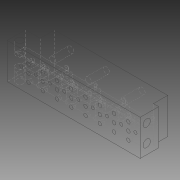
# Autodesk Inventor part: ValveManifold shared no and nc individual common
Saved by Autodesk Inventor 2011 (Build 150239000, 239)
## iProperties
Created: 2012-03-09
Part Number: ValveManifold shared no and nc individual common
Document SubType Name: Modeling
Designer: Marc
Density: 1 g/cm^3
Author: Marc
Autodesk Inventor part; units mm, degrees
ref_plane "YZ Plane" through (0, 0, 0) normal (1, 0, 0) x (0, 1, 0)
ref_plane "XZ Plane" through (0, 0, 0) normal (0, 1, 0) x (-1, 0, 0)
sketch "Sketch1" plane through (0, 0, 0) normal (0, 0, 1) x (1, 0, 0)
  line L0 (0, 0) -> (71.12, 0)
  line L1 (71.12, 0) -> (71.12, 19.05)
  line L2 (71.12, 19.05) -> (0, 19.05)
  line L3 (0, 19.05) -> (0, 0)
  dimension "ManifoldWidth" = 71.12
  dimension "ManifoldDepth" = 19.05
  constraints: 8 end point, 2 parallel, 1 horizontal, 1 perpendicular
  measures "ManifoldWidth" distance of L0.start L0.end
  measures "ManifoldDepth" distance of L0.end L1.end
extrude "Extrusion1" add sketch "Sketch1" along normal blind 17.4625
sketch "hdi facemount placement" plane through (0, 0, 17.4625) normal (0, 0, 1) x (1, 0, 0)
  line L0 (0, 0) -> (0, 19.05) projected
  line L1 (71.12, 0) -> (0, 0) projected
  line L2 (71.12, 19.05) -> (71.12, 0) projected
  line L3 (0, 19.05) -> (71.12, 19.05) projected
  line L4 (11.43, 13.7668) -> (11.43, 5.2832)
  line L5 (7.62, 10.7442) -> (15.24, 10.7442)
  line L6 (35.56, 19.05) -> (35.56, 0)
  line L7 (0, 9.525) -> (71.12, 9.525)
  point P0 (11.43, 9.525)
  point P1 (19.05, 5.2832)
  point P2 (22.86, 10.7442)
  point P3 (19.05, 13.7668)
  point P4 (19.05, 9.525)
  point P5 (26.67, 5.2832)
  point P6 (30.48, 10.7442)
  point P7 (26.67, 13.7668)
  point P8 (26.67, 9.525)
  point P9 (34.29, 5.2832)
  point P10 (38.1, 10.7442)
  point P11 (34.29, 13.7668)
  point P12 (34.29, 9.525)
  point P13 (41.91, 5.2832)
  point P14 (45.72, 10.7442)
  point P15 (41.91, 13.7668)
  point P16 (41.91, 9.525)
  point P17 (49.53, 5.2832)
  point P18 (53.34, 10.7442)
  point P19 (49.53, 13.7668)
  point P20 (49.53, 9.525)
  point P21 (57.15, 5.2832)
  point P22 (60.96, 10.7442)
  point P23 (57.15, 13.7668)
  point P24 (57.15, 9.525)
  point P25 (64.77, 5.2832)
  point P26 (68.58, 10.7442)
  point P27 (64.77, 13.7668)
  point P28 (64.77, 9.525)
  dimension "d4" = 8.4836
  dimension "d5" = 7.62
  dimension "d6" = 3.0226
  dimension "d7" = 1.2192
  dimension "d10" = 7.62
  dimension "d106" = 5.2832
  dimension "d160" = 7.62
  constraints: 8 end point, 5 midpoint, 4 coincident, 2 perpendicular, 1 horizontal, 1 point on line, 1 symmetric about line, 28 other
  measures "d4" distance of L4.start L4.end
  measures "d5" distance of L5.start L5.end
  measures "d6" vertical distance of L4.start L5.end
  measures "d7" distance from line of L5 point (11.43, 9.525)
  measures "d10" distance of point (11.43, 13.767) point (19.05, 13.767)
  measures "d106" distance from line of L3 L4.start
  measures "d160" distance from line of L0 L5.start
hole "facemount tapped holes" at (7.62, 10.7442, 17.4625) at (15.24, 10.7442, 17.4625) at (22.86, 10.7442, 17.4625) at (30.48, 10.7442, 17.4625) at (38.1, 10.7442, 17.4625) at (45.72, 10.7442, 17.4625) at (53.34, 10.7442, 17.4625) at (60.96, 10.7442, 17.4625) at (68.58, 10.7442, 17.4625) direction (0, 0, -1) diameter 1.7018 depth 6.35 tip angle 118
hole "normally open holes" at (11.43, 13.7668, 17.4625) at (19.05, 13.7668, 17.4625) at (26.67, 13.7668, 17.4625) at (34.29, 13.7668, 17.4625) at (41.91, 13.7668, 17.4625) at (49.53, 13.7668, 17.4625) at (57.15, 13.7668, 17.4625) at (64.77, 13.7668, 17.4625) direction (0, 0, -1) diameter 1.9304 depth 3.4417 tip angle 118
hole "normally closed holes" at (11.43, 5.2832, 17.4625) at (19.05, 5.2832, 17.4625) at (26.67, 5.2832, 17.4625) at (34.29, 5.2832, 17.4625) at (41.91, 5.2832, 17.4625) at (49.53, 5.2832, 17.4625) at (57.15, 5.2832, 17.4625) at (64.77, 5.2832, 17.4625) direction (0, 0, -1) diameter 1.9304 depth 3.4417 tip angle 118
hole "shallow common holes" at (11.43, 9.525, 17.4625) at (26.67, 9.525, 17.4625) at (41.91, 9.525, 17.4625) at (57.15, 9.525, 17.4625) direction (0, 0, -1) diameter 1.9304 depth 7.9375 tip angle 118
hole "deep common holes" at (19.05, 9.525, 17.4625) at (34.29, 9.525, 17.4625) at (49.53, 9.525, 17.4625) at (64.77, 9.525, 17.4625) direction (0, 0, -1) diameter 1.9304 depth 13.0175 tip angle 118
sketch "Sketch3" plane through (71.12, 0, 0) normal (1, 0, 0) x (0, 0, -1)
  line L0 (-17.4625, 12.8016) -> (-17.4625, 14.732) projected
  line L1 (0, 0) -> (-17.4625, 0) projected
  line L2 (-17.4625, 0) -> (-17.4625, 19.05) projected
  line L3 (-17.4625, 19.05) -> (0, 19.05) projected
  line L4 (0, 19.05) -> (0, 0) projected
  line L5 (0, 0) -> (-17.4625, 0) projected
  line L6 (-17.4625, 0) -> (-17.4625, 19.05) projected
  line L7 (-17.4625, 19.05) -> (0, 19.05) projected
  line L8 (0, 19.05) -> (0, 0) projected
  line L9 (-14.0208, 14.732) -> (-14.0208, 12.8016) projected
  line L10 (-14.0208, 12.8016) -> (-17.4625, 12.8016) projected
  line L11 (-14.0208, 14.732) -> (-17.4625, 14.732) projected
  line L12 (-14.0208, 6.2484) -> (-17.4625, 6.2484) projected
  line L13 (-14.0208, 4.318) -> (-17.4625, 4.318) projected
  line L14 (-14.0208, 6.2484) -> (-14.0208, 4.318) projected
  line L15 (-11.1125, 11.5951) -> (-17.4625, 11.5951) projected
  line L16 (-10.8458, 7.1163) -> (-10.8458, 3.4501)
  line L17 (-10.8458, 3.4501) -> (-14.0208, 1.617)
  line L18 (-14.0208, 1.617) -> (-17.1958, 3.4501)
  line L19 (-17.1958, 3.4501) -> (-17.1958, 7.1163)
  line L20 (-17.1958, 7.1163) -> (-14.0208, 8.9494)
  line L21 (-14.0208, 8.9494) -> (-10.8458, 7.1163)
  circle A0 centre (-14.0208, 5.2832) radius 3.6662
  line L22 (-10.8458, 16.5651) -> (-10.8458, 12.8989)
  line L23 (-10.8458, 12.8989) -> (-14.0208, 11.0658)
  line L24 (-14.0208, 11.0658) -> (-17.1958, 12.8989)
  line L25 (-17.1958, 12.8989) -> (-17.1958, 16.5651)
  line L26 (-17.1958, 16.5651) -> (-14.0208, 18.3982)
  line L27 (-14.0208, 18.3982) -> (-10.8458, 16.5651)
  circle A1 centre (-14.0208, 14.732) radius 3.6662
  point P0 (-17.4625, 13.7668)
  dimension "d44" = 3.1369
  dimension "d121" = 5.2832
  dimension "d122" = 4.318
  dimension "d161" = 6.35
  dimension "d162" = 9.4488
  constraints: 24 end point, 6 coincident, 2 collinear, 2 vertical alignment, 1 midpoint, 1 parallel, 30 other
  measures "d44" distance from line of L15 L9.start
  measures "d121" distance from line of L1 point (-14.021, 5.283)
  measures "d122" distance from line of L3 L9.start
  measures "d161" distance between parallel lines of L17 L20
  measures "d162" distance of point (-14.021, 14.732) point (-14.021, 5.283)
hole "shared reservoirs" at (71.12, 5.2832, 14.0208) at (71.12, 14.732, 14.0208) direction (-1, 0, 0) diameter 3.9624 depth 67.945 tip angle 118 thread size "10-32 UNF" class "2B" standard "ANSI Unified Screw Threads"
sketch "Sketch6" plane through (0, 0, 0) normal (0, 0, -1) x (-1, 0, 0)
  line L0 (-71.12, 19.05) -> (0, 19.05) projected
  arc A0 (-26.67, 12.8016) -> (-26.67, 12.8016) centre (-26.67, 12.8016) ccw projected
  line L1 (-3.175, 16.7132) -> (-71.12, 16.7132) projected
  arc A1 (-26.67, 4.318) -> (-26.67, 4.318) centre (-26.67, 4.318) ccw projected
  line L2 (-3.175, 3.302) -> (-71.12, 3.302) projected
  line L3 (-3.175, 12.7508) -> (-71.12, 12.7508) projected
  circle A2 centre (-30.48, 10.7442) radius 0.8509 projected
  circle A3 centre (-22.86, 10.7442) radius 0.8509 projected
  line L4 (-35.56, 19.05) -> (-35.56, 0) projected
  point P0 (-16.51, 14.2875)
  point P1 (-35.56, 14.2875)
  point P2 (-54.61, 14.2875)
  dimension "d82" = 19.05
  dimension "d87" = 4.7625
  constraints: 1 horizontal, 1 symmetric about line, 4 other
  measures "d82" distance of point (-16.51, 14.287) point (-35.56, 14.287)
  measures "d87" distance from line of L0 point (-16.51, 14.287)
hole "8-32 mounting holes" at (16.51, 14.2875, 0) at (35.56, 14.2875, 0) at (54.61, 14.2875, 0) direction (0, 0, 1) diameter 3.302 depth 9.525 tip angle 118 thread size "8-32 UNC" class "2B" standard "ANSI Unified Screw Threads"
sketch "Sketch9" plane through (0, 19.05, 0) normal (0, 1, 0) x (1, 0, 0)
  line L0 (71.12, 0) -> (71.12, -17.4625) projected
  line L1 (0, 0) -> (0, -17.4625) projected
  line L2 (6.7691, -11.1125) -> (6.7691, -17.4625) projected
  line L3 (3.175, -12.0396) -> (71.12, -12.0396) projected
  line L4 (3.175, -16.002) -> (71.12, -16.002) projected
  line L5 (3.175, -16.002) -> (3.175, -12.0396)
  line L6 (71.12, -16.002) -> (71.12, -12.0396)
  line L7 (71.12, -14.0208) -> (3.175, -14.0208) construction
  circle A0 centre (3.3846, -14.0208) radius 3.3846
  point P0 (0, -17.4625)
  constraints: 6 end point, 2 midpoint, 1 centre point, 1 coincident, 1 collinear, 1 perpendicular, 1 point on line, 1 tangent, 2 other
hole "normally open connection 2" at (3.3845, 19.05, 14.0208) direction (0, -1, 0) diameter 3.9624 depth 6.35 tip angle 118 thread size "10-32 UNF" class "2B" standard "ANSI Unified Screw Threads"
sketch "Sketch10" plane through (0, 0, 0) normal (0, -1, 0) x (1, 0, 0)
  circle A0 centre (3.3845, 14.0208) radius 1.9812 projected
  line L0 (8.9408, 10.8129) -> (3.3845, 7.605)
  line L1 (3.3845, 7.605) -> (-2.1717, 10.8129)
  line L2 (-2.1717, 10.8129) -> (-2.1717, 17.2287)
  line L3 (-2.1717, 17.2287) -> (3.3845, 20.4366)
  line L4 (3.3845, 20.4366) -> (8.9408, 17.2287)
  line L5 (8.9408, 17.2287) -> (8.9408, 10.8129)
  circle A1 centre (3.3845, 14.0208) radius 6.4158
  dimension "d158" = 11.1125
  constraints: 12 end point, 3 coincident, 1 vertical, 16 other
  measures "d158" distance between parallel lines of L5 L2
hole "normally closed connection 2" at (3.3845, 0, 14.0208) direction (0, 1, 0) diameter 3.9624 depth 7.112 tip angle 118 thread size "10-32 UNF" class "2B" standard "ANSI Unified Screw Threads"
sketch "Sketch11" plane through (0, 0, 0) normal (0, -1, 0) x (1, 0, 0)
  line L0 (71.12, 17.4625) -> (0, 17.4625) projected
  line L1 (12.3952, 9.525) -> (12.3952, 17.4625) projected
  line L2 (10.4648, 9.525) -> (10.4648, 17.4625) projected
  line L3 (18.0848, 4.445) -> (18.0848, 17.4625) projected
  line L4 (20.0152, 4.445) -> (20.0152, 17.4625) projected
  line L5 (12.3952, 9.525) -> (10.4648, 9.525) projected
  line L6 (20.0152, 4.445) -> (18.0848, 4.445) projected
  circle A0 centre (11.43, 9.525) radius 3.175
  point P0 (19.05, 4.445)
  point P1 (26.67, 9.525)
  point P2 (34.29, 4.445)
  point P3 (41.91, 9.525)
  point P4 (49.53, 4.445)
  point P5 (57.15, 9.525)
  point P6 (64.77, 4.445)
  dimension "d139" = 15.24
  dimension "d159" = 6.35
  constraints: 2 midpoint, 1 centre point, 1 coincident, 1 horizontal, 6 other
  measures "d139" distance of point (11.43, 9.525) point (26.67, 9.525)
  measures "d159" diameter of A0
ref_plane "Work Plane1" through (11.43, 9.525, 17.4625) normal (0, -1, 0) x (1, 0, 0)
hole "Hole15" at (11.43, 0, 9.525) at (19.05, 0, 4.445) at (26.67, 0, 9.525) at (34.29, 0, 4.445) at (41.91, 0, 9.525) at (49.53, 0, 4.445) at (57.15, 0, 9.525) at (64.77, 0, 4.445) direction (0, 1, 0) diameter 1.016 depth 9.525
hole "Hole16" at (11.43, 0, 9.525) at (19.05, 0, 4.445) at (26.67, 0, 9.525) at (34.29, 0, 4.445) at (41.91, 0, 9.525) at (49.53, 0, 4.445) at (57.15, 0, 9.525) at (64.77, 0, 4.445) direction (0, 1, 0) diameter 3.9624 depth 6.604 countersink diameter 5.1054 countersink angle 90 thread size "10-32 UNF" class "2B" standard "ANSI Unified Screw Threads"
sketch "Sketch12" plane through (0, 0, 0) normal (0, -1, 0) x (1, 0, 0)
  line L0 (14.859, 9.525) -> (14.859, 0) projected
  line L1 (6.7691, 11.1125) -> (6.7691, 17.4625) projected
  line L2 (7.62, 10.6012) -> (6.7691, 11.1125) projected
  line L3 (0, 0) -> (7.874, 0)
  line L4 (7.874, 0) -> (7.874, 7.62)
  line L5 (7.874, 7.62) -> (0, 7.62)
  line L6 (0, 7.62) -> (0, 0)
  line L7 (71.12, 0) -> (68.326, 0)
  line L8 (68.326, 0) -> (68.326, 7.62)
  line L9 (68.326, 7.62) -> (71.12, 7.62)
  line L10 (71.12, 7.62) -> (71.12, 0)
  dimension "d163" = 7.874
  dimension "d164" = 7.62
  dimension "d165" = 7.62
  dimension "d166" = 2.794
  dimension "d169" = 60.452
  constraints: 16 end point, 4 parallel, 2 horizontal, 2 perpendicular
  measures "d163" distance of L4.end L5.end
  measures "d164" distance of L3.end L4.end
  measures "d165" distance of L7.end L8.end
  measures "d166" distance of L8.end L9.end
  measures "d169" distance between parallel lines of L8 L4
extrude "side cuts" cut sketch "Sketch12" along normal through all both and the other way through all
equation "\"common_depth_short\" = commondepth"
equation "\"commondepth\" = 7.9375"
body "Solid1"
